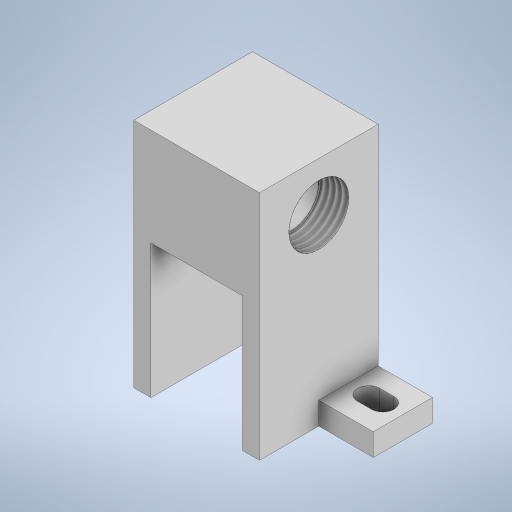
# Autodesk Inventor part: ADAPTER_AOM-brimrose-watercooled-cover
Saved by Autodesk Inventor 2024.2 (Build 282272000, 272)
## iProperties
Created: 2024-02-09
Part Number: ADAPTER_AOM-brimrose-watercooled-cover
Material: Generic
Document SubType Name: Modeling
Designer: fabig
Density: 1 g/cm^3
Appearance: Default
Author: fabig
Autodesk Inventor part; units mm, degrees
ref_plane "YZ Plane" through (0, 0, 0) normal (1, 0, 0) x (0, 1, 0)
ref_plane "XZ Plane" through (0, 0, 0) normal (0, 1, 0) x (-1, 0, 0)
ref_plane "XY Plane" through (0, 0, 0) normal (0, 0, 1) x (1, 0, 0)
sketch "Sketch1" plane through (0, 0, 0) normal (0, 1, 0) x (-1, 0, 0)
  line L0 (-9, 8.5) -> (9, 8.5)
  line L1 (9, 8.5) -> (9, -8.5)
  line L2 (9, -8.5) -> (-9, -8.5)
  line L3 (-9, -8.5) -> (-9, 8.5)
  line L4 (-9, 8.5) -> (9, -8.5) construction
  line L5 (9, 8.5) -> (-9, -8.5) construction
  point P0 (0, 0)
  dimension "d0" = 18
  dimension "d1" = 17
  constraints: 12 end point, 2 midpoint, 2 parallel, 1 horizontal, 1 perpendicular
  measures "d0" distance of L1.end L2.end
  measures "d1" distance of L0.end L1.end
extrude "Extrusion1" add sketch "Sketch1" along normal blind 33.2
sketch "Sketch2" plane through (0, 0, 0) normal (0, -1, 0) x (1, 0, 0)
  line L0 (9, -8.5) -> (-9, -8.5) projected
  line L1 (-6.55, 8.5) -> (6.55, 8.5)
  line L2 (6.55, 8.5) -> (6.55, -8.5)
  line L3 (6.55, -8.5) -> (-6.55, -8.5)
  line L4 (-6.55, -8.5) -> (-6.55, 8.5)
  line L5 (-6.55, 8.5) -> (6.55, -8.5) construction
  line L6 (6.55, 8.5) -> (-6.55, -8.5) construction
  point P0 (0, 0)
  point P1 (-6.55, -8.5)
  dimension "d4" = 13.1
  constraints: 12 end point, 2 midpoint, 2 parallel, 1 horizontal, 1 perpendicular, 1 point on line
  measures "d4" distance of L2.end L3.end
extrude "Extrusion2" cut sketch "Sketch2" against normal blind 19.2
sketch "Sketch4" plane through (0, 0, 0) normal (0, -1, 0) x (1, 0, 0)
  line L0 (9, 8.5) -> (9, -8.5) projected
  line L1 (9, 0) -> (16.8, 0)
  line L2 (16.8, 0) -> (16.8, -8.5)
  line L3 (16.8, -8.5) -> (9, -8.5)
  line L4 (9, -8.5) -> (9, 0)
  line L5 (-9, -8.5) -> (-9, 8.5) projected
  line L6 (-9, -8.5) -> (-16.8, -8.5)
  line L7 (-16.8, -8.5) -> (-16.8, 0)
  line L8 (-16.8, 0) -> (-9, 0)
  line L9 (-9, 0) -> (-9, -8.5)
  point P0 (0, 0)
  dimension "d7" = 7.8
  dimension "d8" = 7.8
  constraints: 16 end point, 4 parallel, 2 horizontal, 2 perpendicular, 1 midpoint, 1 point on line
  measures "d7" distance of L2.end L3.end
  measures "d8" distance of L7.end L8.end
extrude "Extrusion3" add sketch "Sketch4" against normal blind 3.2
sketch "Sketch5" plane through (0, 3.2, 0) normal (0, 1, 0) x (1, 0, 0)
  line L0 (9, 0) -> (9, 8.5) construction
  line L1 (9, 4.25) -> (11.9, 4.25) construction
  circle A0 centre (11.9, 4.25) radius 1.6
  line L2 (11.9, 4.25) -> (13.9, 4.25) construction
  circle A1 centre (13.9, 4.25) radius 1.6
  line L3 (13.9, 5.85) -> (11.9, 5.85)
  line L4 (11.9, 2.65) -> (13.9, 2.65)
  line L5 (-9, 8.5) -> (-9, 0) construction
  line L6 (-9, 4.25) -> (-11.9, 4.25) construction
  line L7 (-11.9, 4.25) -> (-13.9, 4.25) construction
  circle A2 centre (-11.9, 4.25) radius 1.6
  circle A3 centre (-13.9, 4.25) radius 1.6
  line L8 (-13.9, 5.85) -> (-11.9, 5.85)
  line L9 (-13.9, 2.65) -> (-11.9, 2.65)
  point P0 (0, 0)
  dimension "d11" = 2.9
  dimension "d12" = 3.2
  dimension "d13" = 2
  dimension "d14" = 3.2
  dimension "d17" = 2.9
  dimension "d18" = 2
  dimension "d19" = 3.2
  dimension "d20" = 3.2
  constraints: 16 end point, 8 point on circle, 8 tangent, 4 centre point, 4 coincident, 4 horizontal, 2 midpoint
  measures "d11" distance of L1.start L1.end
  measures "d12" diameter of A0
  measures "d13" distance of L2.start L2.end
  measures "d14" diameter of A1
  measures "d17" distance of L6.start L6.end
  measures "d18" distance of L6.end L7.end
  measures "d19" diameter of A2
  measures "d20" diameter of A3
extrude "Extrusion4" cut sketch "Sketch5" against normal through all
sketch "Sketch6" plane through (9, 0, 8.5) normal (1, 0, 0) x (0, 0, -1)
  line L0 (0, 33.2) -> (17, 33.2) construction
  line L1 (8.5, 33.2) -> (8.5, 26.2) construction
  circle A0 centre (8.5, 26.2) radius 4
  point P0 (8.5, 0)
  dimension "d21" = 7
  dimension "d22" = 8
  constraints: 2 end point, 1 centre point, 1 coincident, 1 midpoint, 1 vertical
  measures "d21" distance of L1.start L1.end
  measures "d22" diameter of A0
extrude "Extrusion5" cut sketch "Sketch6" against normal through all
sketch "Sketch8" plane through (9, 0, 8.5) normal (1, 0, 0) x (0, 0, -1)
  line L0 (0, 33.2) -> (17, 33.2) construction
  line L1 (8.5, 33.2) -> (8.5, 26.2) construction
  point P0 (8.5, 0)
  dimension "d33" = 7
  constraints: 2 end point, 1 midpoint, 1 vertical
  measures "d33" distance of L1.start L1.end
hole "Hole2" at (9, 26.2, 0) direction (-1, 0, 0) diameter 8.566 depth 4 thread size "G 1/8-28" standard "BSP Pipe Threads"
sketch "Sketch9" plane through (-9, 0, 8.5) normal (-1, 0, 0) x (0, 0, 1)
  line L0 (-17, 33.2) -> (0, 33.2) construction
  line L1 (-8.5, 33.2) -> (-8.5, 26.2) construction
  point P0 (-8.5, 0)
  dimension "d41" = 7
  constraints: 2 end point, 1 midpoint, 1 vertical
  measures "d41" distance of L1.start L1.end
hole "Hole3" at (-9, 26.2, 0) direction (1, 0, 0) diameter 8.566 depth 4 thread size "G 1/8-28" standard "BSP Pipe Threads"
body "Solid1"
